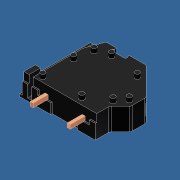
# Autodesk Inventor part: Wago 745-831 (32A) Black
Saved by Autodesk Inventor 2012 (Build 160160000, 160)
## iProperties
Category: PARTsolutions
Company: Team 801
Created: 2007-09-01
Part Number: Wago 745-831 (32A) Black
Catalog Web Link: www.team801.org
Description: 745-831 - MODULAR PCB TERMINAL BLOCK 2 SOLDER PINS / POLE PIN SPACING 7.5 MM / 0.295 IN
Document SubType Name: Modeling
Designer: Jeffrey M
Mass: 3.7945 g
Surface Area: 22.6287 cm^2
Volume: 3.7945 cm^3
Density: 1 g/cm^3
Material: Default
NB: 745-831
NN: 745-831
NT: MODULAR PCB TERMINAL BLOCK 2 SOLDER PINS / POLE PIN SPACING 7.5 MM / 0.295 IN
NBSYN: $BESTNR.
LINA: 745-831
BESTNR: 745-831
QUERSCHNITT1: 0.2 - 6
QUERSCHNITT2: 24 - 10
ABISOLIERLAENGE: 11 - 12
SPANNUNG: 400
BEMESSSTOSSSPG: 6
VERSCHMUTZGRAD: 3
STROM: 32
RM: 7.50
P: 1
HOEHE: 23.00
BREITE: 7.50
TIEFE: 29.10
ANZAHLKLEMMSTEL: 1
ANZAHLPOTENTIAL: 1
FARBE: grau
GEWICHT: 4.760
EAN: 4044918302609
BOHRLOCHDURCHM: 1,8 + 0,1 mm
RGB: 0.67,0.67,0.67,0
KT: DUMMY
PSOL_IDENT_0: {\\partserver001.servicenet\dplatte\cadenas\23d-libs\wago\pg04\serie745\0745-0831_0999-0962.prj},149
PSOL_IDENT_1: {VTYP=3D},{NB=745-831},{LINA=745-831},{NN=745-831},{DATE=10.04.2007 09:25:17},{GEOMDATE=13.06.2006}
PSOL_IDENT_2: ,{VERSION=},{LINEID=160},{LINESUBID=-1},{WBVAR=}  {NB=745-831},{LINA=745-831},{KT=DUMMY},{BESTNR=745
PSOL_IDENT_3: -831},{QUERSCHNITT1=0.2 - 6},{QUERSCHNITT2=24 - 10},{ABISOLIERLAENGE=11 - 12},{SPANNUNG=400},{BEMESS
PSOL_IDENT_4: STOSSSPG=6},{VERSCHMUTZGRAD=3},{STROM=32},{RM=7.50},{P=1},{HOEHE=23.00},{BREITE=7.50},{TIEFE=29.10},
PSOL_IDENT_5: {ANZAHLKLEMMSTEL=1},{ANZAHLPOTENTIAL=1},{FARBE=grau},{GEWICHT=4.760},{EAN=4044918302609},{BOHRLOCHDU
PSOL_IDENT_6: RCHM=1,8 + 0,1 mm},{RGB=0.67,0.67,0.67,0}
Title: Wago 745-831 (32A)
Author: Jeffrey M
Comments: MODULAR PCB TERMINAL BLOCK 2 SOLDER PINS / POLE PIN SPACING 7.5 MM / 0.295 IN
Autodesk Inventor part; units mm, degrees
ref_plane "YZ Plane" through (0, 0, 0) normal (1, 0, 0) x (0, 1, 0)
ref_plane "XZ Plane" through (0, 0, 0) normal (0, 1, 0) x (-1, 0, 0)
ref_plane "XY Plane" through (0, 0, 0) normal (0, 0, 1) x (1, 0, 0)
sketch "Skizze_1" plane through (0, 0, 0) normal (0, 0, 1) x (1, 0, 0)
  line L0 (-20.2, 0) -> (4.4, 0)
  line L1 (4.4, 0) -> (4.4, 4.3858)
  arc A0 (4.6929, 5.0929) -> (4.4, 4.3858) centre (5.4, 4.3858) ccw
  line L2 (4.6929, 5.0929) -> (7.7071, 8.1071)
  arc A1 (7.7071, 8.1071) -> (8, 8.8142) centre (7, 8.8142) ccw
  line L3 (8, 8.8142) -> (8, 13.1387)
  arc A2 (8, 13.1387) -> (7.7071, 13.8458) centre (7, 13.1387) ccw
  line L4 (7.7071, 13.8458) -> (-1.1542, 22.7071)
  arc A3 (-1.1542, 22.7071) -> (-1.8613, 23) centre (-1.8613, 22) ccw
  line L5 (-1.8613, 23) -> (-14.5499, 23)
  arc A4 (-14.5499, 23) -> (-15.0197, 22.671) centre (-14.5499, 22.5) ccw
  line L6 (-15.0197, 22.671) -> (-17.0733, 17.029)
  arc A5 (-17.5431, 16.7) -> (-17.0733, 17.029) centre (-17.5431, 17.2) ccw
  line L7 (-17.5431, 16.7) -> (-17.9972, 16.7)
  arc A6 (-18.4969, 17.1826) -> (-17.9972, 16.7) centre (-17.9972, 17.2) ccw
  line L8 (-18.4969, 17.1826) -> (-18.6899, 22.7105)
  arc A7 (-18.6899, 22.7105) -> (-18.9897, 23) centre (-18.9897, 22.7) ccw
  line L9 (-18.9897, 23) -> (-19.9, 23)
  arc A8 (-19.9, 23) -> (-20.2, 22.7) centre (-19.9, 22.7) ccw
  line L10 (-20.2, 22.7) -> (-20.2, 0)
  constraints: 22 end point, 18 point on circle, 9 centre point
extrude "Extrusion1" add sketch "Skizze_1" along normal blind 7.5
sketch "Skizze_2" plane through (0, 0, 0) normal (0, 0, 1) x (1, 0, 0)
  arc A0 (-11.4012, 22.3457) -> (-11.71, 23) centre (-11.71, 22.6) ccw
  line L0 (-11.4012, 22.3457) -> (-11.5282, 22.1915)
  arc A1 (-11.5282, 22.1915) -> (-11.2475, 21.3998) centre (-11.15, 21.88) ccw
  line L1 (-11.2475, 21.3998) -> (-11.15, 21.38)
  line L2 (-11.15, 21.38) -> (-7.25, 21.38)
  line L3 (-7.25, 21.38) -> (-7.1525, 21.3998)
  arc A2 (-7.1525, 21.3998) -> (-6.8718, 22.1915) centre (-7.25, 21.88) ccw
  line L4 (-6.8718, 22.1915) -> (-6.9988, 22.3457)
  arc A3 (-6.69, 23) -> (-6.9988, 22.3457) centre (-6.69, 22.6) ccw
  line L5 (-6.69, 23) -> (-11.71, 23)
  constraints: 12 end point, 8 point on circle, 4 centre point
extrude "Extrusion2" cut sketch "Skizze_2" along normal blind 7.5
sketch "Skizze_3" plane through (0, 0, 0) normal (0, 0, 1) x (1, 0, 0)
  line L0 (-21.1, 0) -> (-19.2, 0)
  line L1 (-19.2, 0) -> (-19.2, 23)
  line L2 (-19.2, 23) -> (-19.9, 23)
  arc A0 (-19.9, 23) -> (-21.1, 21.8) centre (-19.9, 21.8) ccw
  line L3 (-21.1, 21.8) -> (-21.1, 17.9727)
  line L4 (-21.1, 17.9727) -> (-20.2, 15.5)
  line L5 (-20.2, 15.5) -> (-20.2, 8.5)
  line L6 (-20.2, 8.5) -> (-21.1, 6.0273)
  line L7 (-21.1, 6.0273) -> (-21.1, 0)
  constraints: 16 end point, 2 point on circle, 1 centre point
extrude "Extrusion3" add sketch "Skizze_3" along normal blind 0.8
sketch "Skizze_4" plane through (0, 0, 7.5) normal (0, 0, 1) x (1, 0, 0)
  line L0 (-18.7, 23) -> (-18.4, 14.4091)
  line L1 (-18.4, 14.4091) -> (-18.4, 0)
  line L2 (-18.4, 0) -> (-17, 0)
  line L3 (-17, 0) -> (-17, 23)
  line L4 (-17, 23) -> (-18.7, 23)
  constraints: 10 end point
extrude "Extrusion4" cut sketch "Skizze_4" against normal blind 6.6
sketch "Skizze_5" plane through (0, 0, 7.5) normal (0, 0, 1) x (1, 0, 0)
  line L0 (-20.2, 4.4) -> (-18.4, 4.4)
  line L1 (-18.4, 4.4) -> (-18.4, 27.4)
  line L2 (-18.4, 27.4) -> (-20.2, 27.4)
  line L3 (-20.2, 27.4) -> (-20.2, 4.4)
  constraints: 8 end point
extrude "Extrusion5" cut sketch "Skizze_5" against normal blind 2.8
sketch "Skizze_7" plane through (0, 0, 7.5) normal (0, 0, 1) x (1, 0, 0)
  line L0 (-19.4, 23) -> (-19.4, 21.5)
  line L1 (-19.4, 21.5) -> (-18.4, 21.5)
  line L2 (-18.4, 21.5) -> (-18.4, 23)
  line L3 (-18.4, 23) -> (-19.4, 23)
  constraints: 8 end point
extrude "Extrusion6" cut sketch "Skizze_7" against normal blind 6.3
sketch "Skizze_8" plane through (0, 0, 7.5) normal (0, 0, 1) x (1, 0, 0)
  circle A0 centre (6.2, 9.7) radius 0.8
  constraints: 1 centre point
extrude "Extrusion7" add sketch "Skizze_8" along normal blind 1.5
sketch "Skizze_9" plane through (0, 0, 7.5) normal (0, 0, 1) x (1, 0, 0)
  circle A0 centre (3.7, 6.7) radius 0.8
  constraints: 1 centre point
extrude "Extrusion8" add sketch "Skizze_9" along normal blind 1.5
sketch "Skizze_10" plane through (0, 0, 7.5) normal (0, 0, 1) x (1, 0, 0)
  circle A0 centre (-2.5, 2.4) radius 0.8
  constraints: 1 centre point
extrude "Extrusion9" add sketch "Skizze_10" along normal blind 1.5
sketch "Skizze_11" plane through (0, 0, 7.5) normal (0, 0, 1) x (1, 0, 0)
  circle A0 centre (-15.2, 1.9) radius 0.8
  constraints: 1 centre point
extrude "Extrusion10" add sketch "Skizze_11" along normal blind 1.5
sketch "Skizze_12" plane through (0, 0, 7.5) normal (0, 0, 1) x (1, 0, 0)
  circle A0 centre (-15.2, 12.3) radius 0.8
  constraints: 1 centre point
extrude "Extrusion11" add sketch "Skizze_12" along normal blind 1.5
sketch "Skizze_13" plane through (0, 0, 7.5) normal (0, 0, 1) x (1, 0, 0)
  circle A0 centre (-14.1, 18.1) radius 0.8
  constraints: 1 centre point
extrude "Extrusion12" add sketch "Skizze_13" along normal blind 1.5
sketch "Skizze_14" plane through (0, 0, 7.5) normal (0, 0, 1) x (1, 0, 0)
  circle A0 centre (-9.7, 19.6) radius 0.8
  constraints: 1 centre point
extrude "Extrusion13" add sketch "Skizze_14" along normal blind 1.5
sketch "Skizze_15" plane through (0, 0, 7.5) normal (0, 0, 1) x (1, 0, 0)
  circle A0 centre (0.7, 17.9) radius 0.8
  constraints: 1 centre point
extrude "Extrusion14" add sketch "Skizze_15" along normal blind 1.5
sketch "Skizze_6" plane through (0, 0, 2.4) normal (0, 0, 1) x (1, 0, 0)
  arc A0 (-17.2598, 21.95) -> (-17, 21.5) centre (-17, 21.8) ccw
  line L0 (-17, 21.5) -> (-17, 16.5)
  line L1 (-17, 16.5) -> (-13.9, 16.5)
  line L2 (-13.9, 16.5) -> (-13.9, 23)
  line L3 (-13.9, 23) -> (-16.3649, 23)
  arc A1 (-16.3649, 23) -> (-16.7979, 22.75) centre (-16.3649, 22.5) ccw
  line L4 (-16.7979, 22.75) -> (-17.2598, 21.95)
  constraints: 10 end point, 4 point on circle, 2 centre point
extrude "Extrusion15" add sketch "Skizze_6" along normal blind 3.5
sketch "Skizze_16" plane through (0, 0, 0) normal (0, 1, 0) x (-1, 0, 0)
  line L0 (20.2, 4.9) -> (20.2, 7.5)
  line L1 (20.2, 7.5) -> (-4.4, 7.5)
  line L2 (-4.4, 7.5) -> (-4.4, 4.9)
  line L3 (-4.4, 4.9) -> (-2.4, 4.9)
  line L4 (-2.4, 4.9) -> (-2.4, 3.4)
  line L5 (-2.4, 3.4) -> (1.6, 3.4)
  line L6 (1.6, 3.4) -> (1.6, 0)
  line L7 (1.6, 0) -> (10.6, 0)
  line L8 (10.6, 0) -> (10.6, 3.4)
  line L9 (10.6, 3.4) -> (15, 3.4)
  line L10 (15, 3.4) -> (15, 4.9)
  line L11 (15, 4.9) -> (17, 4.9)
  line L12 (17, 4.9) -> (17, 2.8)
  line L13 (17, 2.8) -> (18.4, 2.8)
  line L14 (18.4, 2.8) -> (18.4, 4.9)
  line L15 (18.4, 4.9) -> (20.2, 4.9)
  constraints: 32 end point
extrude "Extrusion16" cut sketch "Skizze_16" along normal blind 0.5
sketch "Skizze_17" plane through (0, 0, 0) normal (0, 1, 0) x (-1, 0, 0)
  line L0 (0.5, 3.45) -> (0.5, 4.85)
  line L1 (0.5, 4.85) -> (-0.5, 4.85)
  line L2 (-0.5, 4.85) -> (-0.5, 3.45)
  line L3 (-0.5, 3.45) -> (0.5, 3.45)
  constraints: 8 end point
extrude "Extrusion17" add sketch "Skizze_17" along normal mid plane 9
pattern_linear "Rectangular Pattern1" count 2 spacing 12.5 along (-1, 0, 0) of "Extrusion17"
sketch "Skizze_19" plane through (0, 0, 3.75) normal (0, 0, 1) x (1, 0, 0)
  line L0 (4.2704, 14.4541) -> (5.6846, 15.8683)
  line L1 (5.6846, 15.8683) -> (8.2302, 13.3227)
  line L2 (8.2302, 13.3227) -> (7.6506, 13.1674)
  line L3 (7.6506, 13.1674) -> (6.6038, 12.1206)
  line L4 (6.6038, 12.1206) -> (4.2704, 14.4541)
  line L5 (4.2704, 14.4541) -> (5.6846, 15.8683)
  constraints: 12 end point
revolve "Revolution1" cut sketch "Skizze_19" angle 360 about axis through (4.2704, 14.4541, 3.75) along (-0.7071, -0.7071, 0)
sketch "Skizze_20" plane through (0, 0, 4.5) normal (0, 0, 1) x (1, 0, 0)
  line L0 (1.8662, 19.6867) -> (0.452, 18.2725)
  line L1 (0.452, 18.2725) -> (-0.3612, 19.0856)
  line L2 (-0.3612, 19.0856) -> (0.6244, 20.0712)
  line L3 (0.6244, 20.0712) -> (0.8056, 20.7473)
  line L4 (0.8056, 20.7473) -> (1.8662, 19.6867)
  line L5 (1.8662, 19.6867) -> (0.452, 18.2725)
  constraints: 12 end point
revolve "Revolution2" cut sketch "Skizze_20" angle 360 about axis through (1.8662, 19.6867, 4.5) along (0.7071, 0.7071, 0)
sketch "Skizze_21" plane through (0, 0, 0.9) normal (0, 0, 1) x (1, 0, 0)
  line L0 (-5.5179, 21) -> (-2.2755, 21)
  line L1 (-2.2755, 21) -> (-0.644, 19.3685)
  line L2 (-0.644, 19.3685) -> (0.7702, 20.7827)
  line L3 (0.7702, 20.7827) -> (-1.4471, 23)
  line L4 (-1.4471, 23) -> (-4.4836, 23)
  arc A0 (-4.2007, 22.3172) -> (-4.4836, 23) centre (-4.4836, 22.6) ccw
  line L5 (-4.2007, 22.3172) -> (-5.5179, 21)
  constraints: 12 end point, 2 point on circle, 1 centre point
extrude "Extrusion18" cut sketch "Skizze_21" along normal blind 5.8
sketch "Sketch21" plane through (4.2704, 14.4541, 3.75) normal (0.7071, 0.7071, 0) x (-0.7071, 0.7071, 0)
  circle A0 centre (0, 0) radius 3.3 projected
body "Solid1"
